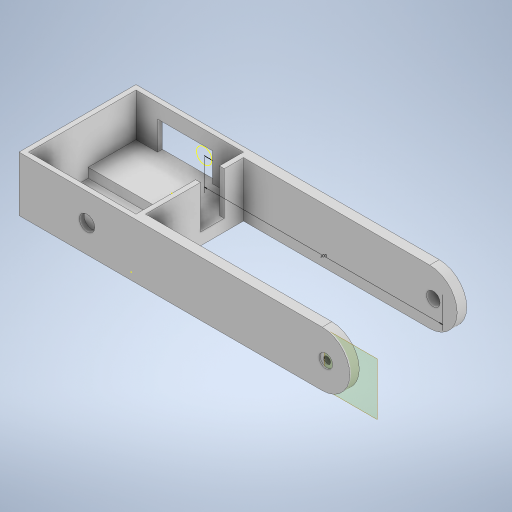
# Autodesk Inventor part: servo_box
Saved by Autodesk Inventor 2024.3 (Build 283343000, 343)
## iProperties
Created: 2024-07-16
Part Number: servo_box
Material: Ogólny
Document SubType Name: Modeling
Designer: User
Density: 1 g/cm^3
Appearance: Domyślna
Author: User
Autodesk Inventor part; units mm, degrees
ref_plane "YZ Plane" through (0, 0, 0) normal (1, 0, 0) x (0, 1, 0)
ref_plane "XZ Plane" through (0, 0, 0) normal (0, 1, 0) x (-1, 0, 0)
ref_plane "XY Plane" through (0, 0, 0) normal (0, 0, 1) x (1, 0, 0)
sketch "Szkic1" plane through (0, 0, 0) normal (0, 1, 0) x (-1, 0, 0)
  line L0 (0, 0) -> (45, 0)
  line L1 (45, 0) -> (45, -30)
  line L2 (45, -30) -> (0, -30)
  line L3 (0, -30) -> (0, 0)
  line L4 (45, 0) -> (45, 2)
  line L5 (45, 2) -> (47, 2)
  line L6 (0, -30) -> (0, -32)
  line L7 (0, -32) -> (-2, -32)
  line L8 (-2, -32) -> (47, -32)
  line L9 (47, -32) -> (47, 2)
  line L10 (47, 2) -> (-2, 2)
  line L11 (-2, 2) -> (-2, -32)
  line L12 (47, 2) -> (47, 17)
  line L13 (-2, 2) -> (-2, 17)
  line L14 (-2, 17) -> (47, 17)
  line L15 (-2, 17) -> (-2, 15)
  line L16 (-2, 15) -> (47, 15)
  line L17 (47, 17) -> (47, 14.5669)
  line L18 (0, 2) -> (0, 15)
  line L19 (45, 2) -> (45, 15)
  line L20 (0, 0) -> (0, 2)
  line L21 (45, 0) -> (45, 2)
  dimension "d0" = 45
  dimension "d1" = 30
  dimension "d2" = 2
  dimension "d3" = 2
  dimension "d4" = 2
  dimension "d5" = 2
  dimension "d40" = 15
  dimension "d41" = 15
  dimension "d42" = 2
  constraints: 44 end point, 7 perpendicular, 6 point on line, 5 parallel, 4 vertical, 2 horizontal, 1 collinear
  measures "d0" distance of L1.end L2.end
  measures "d1" distance of L0.end L1.end
  measures "d2" distance of L0.end L4.end
  measures "d3" distance of L4.end L5.end
  measures "d4" distance of L2.end L6.end
  measures "d5" distance of L6.end L7.end
  measures "d40" distance of L5.end L12.end
  measures "d41" distance of L10.end L13.end
  measures "d42" distance of L13.end L15.end
extrude "Wyciągnięcie proste1" add sketch "Szkic1" along normal blind 20 contours L3 L6 L7 L11 L10 L20 | L4 L5 L9 L8 L6 L2 L1 | L10 L13 L16 L18 | L19 L16 L12 L5 | L16 L13 L14 L12
sketch "Szkic2" plane through (0, 0, 0) normal (0, -1, 0) x (1, 0, 0)
  line L0 (-47, 2) -> (2, 2) projected
  line L1 (-47, -32) -> (-47, 17) projected
  line L2 (2, 2) -> (-47, 2)
  line L3 (-47, 2) -> (-47, -32)
  line L4 (-47, -32) -> (2, -32)
  line L5 (2, -32) -> (2, 2)
  point P0 (0, 0)
  constraints: 8 end point, 2 parallel, 1 horizontal, 1 perpendicular
extrude "Wyciągnięcie proste2" add sketch "Szkic2" against normal blind 2
sketch "Szkic3" plane through (2, 0, -32) normal (0, 0, -1) x (-1, 0, 0)
  line L0 (40, 2) -> (15, 2)
  line L1 (15, 2) -> (15, 14)
  line L2 (15, 14) -> (40, 14)
  line L3 (40, 14) -> (40, 2)
  line L4 (40, 14) -> (38, 14)
  line L5 (38, 14) -> (38, 2)
  line L6 (38, 2) -> (40, 2)
  line L7 (40, 2) -> (40, 14)
  point P0 (2, 0)
  dimension "d10" = 25
  dimension "d11" = 12
  dimension "d30" = 2
  constraints: 16 end point, 4 parallel, 2 horizontal, 2 perpendicular, 1 point on line
  measures "d10" distance of L1.end L2.end
  measures "d11" distance of L0.end L1.end
  measures "d30" distance of L6.end L5.end
extrude "Wyciągnięcie proste3" cut sketch "Szkic3" against normal blind 4.5 contours L0 L1 L2 L5
sketch "Szkic4" plane through (0, 20, 0) normal (0, 0, -1) x (-1, 0, 0)
  line L0 (38, -6) -> (38, -18) projected
  line L1 (38, -12) -> (28, -12)
  line L2 (28, -12) -> (30.5, -12)
  circle A0 centre (30.5, -12) radius 4.5
  line L3 (13, -6) -> (36, -6) projected
  line L4 (24.5, -6) -> (24.5, -18)
  line L5 (0, -18) -> (45, -18) projected
  line L6 (11, -12) -> (21, -12)
  circle A1 centre (18.5, -12) radius 4.5
  point P0 (0, -20)
  dimension "d14" = 10
  dimension "d15" = 2.5
  dimension "d16" = 9
  constraints: 8 end point, 4 symmetric about line, 3 point on line, 2 centre point, 2 coincident, 2 midpoint, 1 horizontal, 1 vertical, 1 other
  measures "d14" distance of L1.start L1.end
  measures "d15" distance of L1.end L2.end
  measures "d16" diameter of A0
extrude "Wyciągnięcie proste4" [suppressed]
sketch "Szkic5" plane through (0, 20, 0) normal (0, 1, 0) x (1, 0, 0)
  line L0 (0, 30) -> (0, 0) projected
  line L1 (2, -17) -> (2, 32) projected
  line L2 (0, 9.9645) -> (2, 9.9645)
  line L3 (2, 9.9645) -> (2, 19.9645)
  line L4 (2, 19.9645) -> (0, 19.9645)
  line L5 (0, 19.9645) -> (0, 9.9645)
  point P0 (2, -2)
  dimension "d19" = 10
  constraints: 8 end point, 2 parallel, 2 point on line, 1 horizontal, 1 perpendicular
  measures "d19" distance of L3.end L2.end
extrude "Wyciągnięcie proste5" cut sketch "Szkic5" against normal blind 18
sketch "Szkic6" plane through (-47, 0, 2) normal (0, 0, 1) x (1, 0, 0)
  circle A0 centre (28.5, 8) radius 4.5 projected
  line L0 (28.5, 8) -> (28.5, -2)
  circle A1 centre (28.5, 8) radius 3.5
  circle A2 centre (28.5, 8) radius 4.5
  point P0 (47, 0)
  dimension "d22" = 10
  dimension "d27" = 7
  constraints: 2 centre point, 2 coincident, 2 end point, 1 concentric, 1 vertical
  measures "d22" distance of L0.start L0.end
  measures "d27" diameter of A1
sketch "Szkic7" plane through (0, 0, 0) normal (0, -1, 0) x (1, 0, 0)
  line L0 (2, 17) -> (2, -32) projected
  line L1 (-47, -32) -> (2, -32)
  line L2 (2, -32) -> (2, 2)
  line L3 (2, 2) -> (-47, 2)
  line L4 (-47, 2) -> (-47, -32)
  line L5 (-47, 17) -> (2, 17) projected
  line L6 (-47, 0) -> (2, 0)
  line L7 (2, 0) -> (2, 17)
  line L8 (2, 17) -> (-47, 17)
  line L9 (-47, 17) -> (-47, 0)
  point P0 (0, 0)
  constraints: 16 end point, 4 parallel, 2 horizontal, 2 perpendicular, 1 point on line
extrude "Wyciągnięcie proste6" add sketch "Szkic7" along normal blind 3
sketch "Szkic8" plane through (0, 2, 0) normal (0, 1, 0) x (1, 0, 0)
  line L0 (-45, -2) -> (-45, 30) projected
  line L1 (0, 9.9645) -> (0, 0) projected
  line L2 (-45, 0) -> (0, 0)
  line L3 (0, 0) -> (0, 9.9645)
  line L4 (0, 9.9645) -> (-45, 9.9645)
  line L5 (-45, 9.9645) -> (-45, 0)
  constraints: 8 end point, 2 parallel, 1 horizontal, 1 perpendicular
extrude "Wyciągnięcie proste7" cut sketch "Szkic8" against normal blind 4
extrude "Wyciągnięcie proste8" [suppressed]
sketch "Szkic9" plane through (2, 20, -32) normal (0, 0, -1) x (-1, 0, 0)
  line L0 (15, -6) -> (15, -18) projected
  line L1 (15, -12) -> (20.5, -12)
  circle A0 centre (20.5, -12) radius 3.5
  line L2 (0, -20) -> (0, -23) projected
  line L3 (0, -11.5) -> (29.45, -11.5)
  line L4 (0, -11.5) -> (23.29, -11.5)
  line L5 (23.29, -11.5) -> (20.94, -11.5)
  line L6 (20.94, -11.5) -> (20.94, -12)
  circle A1 centre (20.94, -12) radius 3.5
  point P0 (2, -20)
  point P1 (0, 0)
  dimension "d31" = 5.5
  dimension "d32" = 7
  dimension "d35" = 29.45
  dimension "d36" = 23.29
  dimension "d37" = 2.35
  dimension "d38" = 7
  constraints: 10 end point, 3 point on line, 2 centre point, 2 coincident, 2 horizontal, 1 midpoint, 1 vertical
  measures "d31" distance of L1.start L1.end
  measures "d32" diameter of A0
  measures "d35" distance of L3.start L3.end
  measures "d36" distance of L3.start L4.end
  measures "d37" distance of L4.end L5.end
  measures "d38" diameter of A1
extrude "Wyciągnięcie proste9" cut sketch "Szkic9" against normal blind 47.25 contours A1 L3 A0 | A0 L3 A1 | L3 A0 A1 | A0 L3 A1 picked at (24.181, -11.2212) picked at (22.5407, -11.0097) picked at (22.6367, -12.1539) picked at (24.2617, -12.2698)
sketch "Szkic11" plane through (0, -2, 0) normal (0, 1, 0) x (1, 0, 0)
  line L0 (0, -15) -> (-45, -15) projected
  line L1 (-45, 9.9645) -> (-45, 30) projected
  line L2 (0, -15) -> (-45, -15)
  line L3 (-45, -15) -> (-45, 9.9645)
  line L4 (-45, 9.9645) -> (0, 9.9645)
  line L5 (0, 9.9645) -> (0, -15)
  point P0 (0, 0)
  constraints: 8 end point, 2 parallel, 1 horizontal, 1 perpendicular
extrude "Wyciągnięcie proste10" cut sketch "Szkic11" along normal blind 43.5
sketch "Szkic12" plane through (-18.94, 8, 15.25) normal (0, 0, -1) x (-1, 0, 0)
  point P0 (-18.94, -8)
sketch "Szkic14" plane through (2, 20, -32) normal (0, 0, -1) x (-1, 0, 0)
  line L0 (0, -23) -> (0, 0) projected
  line L1 (0, -11.5) -> (29.51, -11.5)
  line L2 (0, -11.5) -> (29.51, -11.5) construction
  line L3 (29.51, -11.5) -> (18.2, -11.5)
  line L4 (18.2, -11.5) -> (20.515, -11.5)
  circle A0 centre (20.515, -11.5) radius 3.25
  point P0 (2, -20)
  dimension "d47" = 29.51
  dimension "d48" = 0
  dimension "d49" = 11.31
  dimension "d50" = 2.315
  dimension "d51" = 6.5
  constraints: 8 end point, 2 horizontal, 2 point on line, 1 centre point, 1 coincident, 1 collinear, 1 midpoint
  measures "d47" distance of L1.start L1.end
  measures "d48" distance between parallel lines of L1 L2
  measures "d49" distance of L1.end L3.end
  measures "d50" distance of L3.end L4.end
  measures "d51" diameter of A0
extrude "Wyciągnięcie proste11" cut sketch "Szkic14" against normal through all
sketch "Szkic15" plane through (0, 20, 15) normal (0, 0, -1) x (-1, 0, 0)
  arc A0 (20.2611, -8.7589) -> (15.5284, -12.7817) centre (18.515, -11.5) ccw projected
  circle A1 centre (18.515, -11.5) radius 3.25
  arc A2 (15.5284, -12.7817) -> (20.2611, -8.7589) centre (18.94, -12) ccw
  arc A3 (15.5284, -12.7817) -> (20.2611, -8.7589) centre (18.94, -12) ccw projected
  point P0 (0, -20)
  point P1 (15.5284, -12.7817)
  constraints: 2 centre point, 2 point on circle, 1 coincident, 1 concentric
extrude "Wyciągnięcie proste12" add sketch "Szkic15" against normal blind 2 contours A2 A1
sketch "Szkic16" plane through (2, 2, -9.9645) normal (1, 0, 0) x (0, 0, -1)
  line L0 (22.0355, 18) -> (22.0355, -5) projected
  line L1 (22.0355, -5) -> (-26.9645, -5) projected
  line L2 (22.0355, 18) -> (18.0355, 18)
  line L3 (18.0355, 18) -> (18.0355, -5)
  line L4 (18.0355, -5) -> (22.0355, -5)
  line L5 (22.0355, -5) -> (22.0355, 18)
  line L6 (-26.9645, 18) -> (-22.9645, 18)
  line L7 (-22.9645, 18) -> (-22.9645, -5)
  line L8 (-22.9645, -5) -> (-26.9645, -5)
  line L9 (-26.9645, -5) -> (-26.9645, 18)
  point P0 (-9.9645, -2)
  point P1 (-22.9645, -5)
  dimension "d56" = 4
  dimension "d57" = 4
  constraints: 16 end point, 4 parallel, 3 point on line, 2 horizontal, 2 perpendicular
  measures "d56" distance of L4.end L3.end
  measures "d57" distance of L7.end L8.end
sketch "Szkic17" plane through (2, 20, -32) normal (0, 0, -1) x (-1, 0, 0)
  circle A0 centre (20.515, -11.5) radius 3.25 projected
  line L0 (20.515, -11.5) -> (-79.485, -11.5)
  point P0 (2, -20)
  dimension "d58" = 100
  constraints: 2 end point, 1 horizontal
  measures "d58" distance of L0.start L0.end
extrude "Wyciągnięcie proste13" add sketch "Szkic16" along normal blind 79.5
sketch "Szkic18" plane through (-47, -3, -32) normal (0, 0, -1) x (-1, 0, 0)
  line L0 (-128.5, 0) -> (-128.5, 23) projected
  circle A0 centre (-128.5, 11.5) radius 2.85
  line L1 (-128.5, 11.5) -> (-118.5, 11.5)
  line L2 (-118.5, 11.5) -> (-118.5, 5)
  line L3 (-118.5, 5) -> (-146.5, 5)
  line L4 (-146.5, 18) -> (-118.5, 18)
  line L5 (-118.5, 18) -> (-118.5, 11.5)
  line L6 (-128.5, 18) -> (-128.5, 5)
  line L7 (-138.5, 11.5) -> (-138.5, 5)
  line L8 (-138.5, 5) -> (-110.5, 5)
  line L9 (-110.5, 5) -> (-110.5, 18)
  line L10 (-110.5, 18) -> (-138.5, 18)
  line L11 (-138.5, 18) -> (-138.5, 11.5)
  point P0 (-47, 3)
  dimension "d61" = 5.7
  dimension "d62" = 10
  dimension "d63" = 6.5
  dimension "d64" = 28
  dimension "d65" = 13
  constraints: 22 end point, 6 point on line, 5 symmetric about line, 2 perpendicular, 1 centre point, 1 horizontal, 1 midpoint, 1 vertical
  measures "d61" diameter of A0
  measures "d62" distance of L1.start L1.end
  measures "d63" distance of L1.end L2.end
  measures "d64" distance of L2.end L3.end
  measures "d65" distance of L3.end L4.start
sketch "Szkic19" plane through (81.5, 2, -9.9645) normal (1, 0, 0) x (0, 0, -1)
  line L0 (-26.9645, -5) -> (-26.9645, 18) projected
  line L1 (-26.9645, -5) -> (22.0355, -5) projected
  line L2 (-26.9645, 18) -> (-22.9645, 18)
  line L3 (-22.9645, 18) -> (-22.9645, -5)
  line L4 (-22.9645, -5) -> (-26.9645, -5)
  line L5 (-26.9645, -5) -> (-26.9645, 18)
  line L6 (22.0355, 18) -> (18.0355, 18)
  line L7 (18.0355, 18) -> (18.0355, -5)
  line L8 (18.0355, -5) -> (22.0355, -5)
  line L9 (22.0355, -5) -> (22.0355, 18)
  point P0 (-9.9645, -2)
  dimension "d66" = 4
  dimension "d67" = 4
  constraints: 16 end point, 4 parallel, 3 point on line, 2 horizontal, 2 perpendicular
  measures "d66" distance of L3.end L4.end
  measures "d67" distance of L8.end L7.end
extrude "Wyciągnięcie proste14" add sketch "Szkic19" along normal blind 10
extrude "Wyciągnięcie proste15" cut sketch "Szkic18" against normal blind 11.5 contours A0 L0 | L0 L1 A0 | L0 A0 L1
sketch "Szkic20" plane through (-47, -3, 17) normal (0, 0, 1) x (1, 0, 0)
  point P0 (47, 3)
sketch "Szkic21" plane through (-47, -3, 17) normal (0, 0, 1) x (1, 0, 0)
  circle A0 centre (128.5, 11.5) radius 2.85 projected
  circle A1 centre (128.5, 11.5) radius 2.95
  point P0 (47, 3)
  dimension "d72" = 5.9
  constraints: 1 centre point, 1 coincident
  measures "d72" diameter of A1
extrude "Wyciągnięcie proste16" cut sketch "Szkic21" against normal blind 25.25 contours A0
fillet "Zaokrąglenie1" radius 11.5 4 edges at (91.5, 20, -30) (91.5, -3, -30) (91.5, 20, 15) (91.5, -3, 15)
ref_plane "Płaszczyzna konstrukcyjna2" through (91.5, 8.5, 16.5) normal (0, 0, -1) x (-1, 0, 0)
ref_plane "Płaszczyzna konstrukcyjna1" through (91.5, 8.5, 17) normal (0, 0, -1) x (-1, 0, 0)
sketch "Szkic22" plane through (91.5, 8.5, 16.5) normal (0, 0, -1) x (-1, 0, 0)
  circle A0 centre (10, 0) radius 2.85 projected
  circle A1 centre (10, 0) radius 1.5
  circle A2 centre (10, 0) radius 2.85
  point P0 (91.5, -8.5)
  dimension "d77" = 3
  constraints: 2 centre point, 2 coincident
  measures "d77" diameter of A1
extrude "Wyciągnięcie proste17" add sketch "Szkic22" along normal blind 0.25
sketch "Szkic23" plane through (0, 20, 0) normal (0, 1, 0) x (1, 0, 0)
  point P0 (0, 0)
